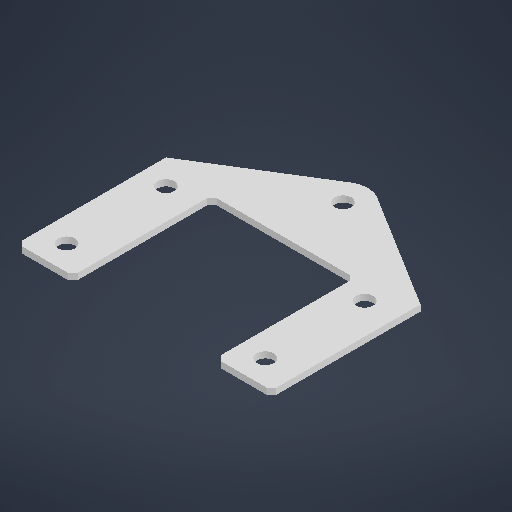
# Autodesk Inventor part: frontFunnel
Saved by Autodesk Inventor 2025.2 (Build 292293000, 293)
## iProperties
Created: 2025-03-23
Part Number: frontFunnel
Material: Generic
Document SubType Name: Modeling
Designer: Jahan
Density: 1 g/cm^3
Appearance: Default
Author: Jahan
Autodesk Inventor part; units mm, degrees
ref_plane "YZ Plane" through (0, 0, 0) normal (1, 0, 0) x (0, 1, 0)
ref_plane "XZ Plane" through (0, 0, 0) normal (0, 1, 0) x (-1, 0, 0)
ref_plane "XY Plane" through (0, 0, 0) normal (0, 0, 1) x (1, 0, 0)
sketch "Sketch1" plane through (0, 0, 0) normal (0, 1, 0) x (-1, 0, 0)
  circle A0 centre (21.6608, 3.3771) radius 2.1844
  circle A1 centre (21.6608, 28.7771) radius 2.1844
  circle A2 centre (-29.1392, 28.7771) radius 2.1844
  circle A3 centre (-29.1392, 3.3771) radius 2.1844
  line L0 (28.0108, 8.7873) -> (28.0108, -1.9569)
  line L1 (21.6608, 35.1271) -> (26.7408, 35.1271)
  line L2 (28.0108, 33.8571) -> (28.0108, -1.9569)
  line L3 (21.6608, 35.1271) -> (14.9933, 35.1271)
  line L4 (26.7408, 35.1271) -> (28.0108, 33.8571)
  line L5 (13.7233, 33.8571) -> (13.7233, 0.8371)
  line L6 (12.4533, -0.4329) -> (-21.5192, -0.4329)
  line L7 (14.9933, 35.1271) -> (13.7233, 33.8571)
  line L8 (13.7233, 0.8371) -> (12.4533, -0.4329)
  line L9 (-22.7892, 0.8371) -> (-22.7892, 33.8571)
  line L10 (-24.0592, 35.1271) -> (-35.8067, 35.1271)
  line L11 (-37.0767, 33.8571) -> (-37.0767, -2.9729)
  line L12 (-22.7892, 33.8571) -> (-24.0592, 35.1271)
  line L13 (-35.8067, 35.1271) -> (-37.0767, 33.8571)
  line L14 (-21.5192, -0.4329) -> (-22.7892, 0.8371)
  line L15 (28.0108, -1.9569) -> (28.0108, 3.3771)
  line L16 (21.6608, 3.3771) -> (47.0608, 3.3771) construction
  line L17 (-37.0767, -2.9729) -> (-7.8315, -21.1135)
  line L18 (28.0108, -1.9569) -> (28.0108, -2.9729)
  line L19 (28.0108, -2.9729) -> (-1.2009, -21.0641)
  arc A4 (-7.8315, -21.1135) -> (-1.2009, -21.0641) centre (-4.5565, -15.6732) ccw
  line L20 (28.0108, -2.9729) -> (-37.0767, -2.9729)
  line L21 (-4.5093, -22.023) -> (-4.5329, -2.9729)
  circle A5 centre (-4.5565, -15.6732) radius 2.1844
  point P0 (0, 0)
  point P1 (28.0108, 35.1271)
  point P2 (13.7233, 35.1271)
  point P3 (13.7233, -0.4329)
  point P4 (-22.7892, -0.4329)
  point P5 (-22.7892, 35.1271)
  point P6 (-37.0767, 35.1271)
  dimension "d0" = 6.35
  dimension "d1" = 1.27
  dimension "d2" = 1.27
  dimension "d3" = 35.56
  dimension "d4" = 1.27
  dimension "d5" = 1.27
  dimension "d6" = 1.27
  dimension "d7" = 1.27
  dimension "d8" = 35.56
  dimension "d9" = 1.27
  dimension "d10" = 1.27
  dimension "d11" = 1.27
  dimension "d12" = 1.27
  dimension "d13" = 1.27
  dimension "d14" = 1.27
  dimension "d18" = 6.35
  dimension "d19" = 1.016
  dimension "d20" = 36.83
  dimension "d21" = 4.3688
  constraints: 44 end point, 13 point on line, 6 centre point, 3 point on circle, 3 vertical, 2 horizontal, 2 perpendicular, 1 coincident, 1 collinear, 1 midpoint, 1 other
  measures "d0" distance of A1.centre L1.start
  measures "d1" distance of L1.end point (28.011, 35.127)
  measures "d2" distance of L2.start point (28.011, 35.127)
  measures "d3" distance of point (13.723, 35.127) point (13.723, -0.433)
  measures "d4" distance of L7.start point (13.723, 35.127)
  measures "d5" distance of L5.start point (13.723, 35.127)
  measures "d6" distance of L5.end point (13.723, -0.433)
  measures "d7" distance of L6.start point (13.723, -0.433)
  measures "d8" distance of point (-22.789, -0.433) point (-22.789, 35.127)
  measures "d9" distance of L9.end point (-22.789, 35.127)
  measures "d10" distance of L12.end point (-22.789, 35.127)
  measures "d11" distance of L13.start point (-37.077, 35.127)
  measures "d12" distance of L11.start point (-37.077, 35.127)
  measures "d13" distance of L14.start point (-22.789, -0.433)
  measures "d14" distance of L9.start point (-22.789, -0.433)
  measures "d18" radius of A4
  measures "d19" distance of L0.end L18.end
  measures "d20" distance of L11.start L11.end
  measures "d21" diameter of A5
extrude "Extrusion1" add sketch "Sketch1" along normal blind 1.5875 contours L0 L18 L20 L11 L13 L10 L12 L9 L14 L6 L8 L5 L7 L3 L1 L4 L2 | L19 A4 L21 A5 L20 | L21 A5 A4 L17 L20
equation "\"d5\" = d4"
equation "\"d6\" = d4"
equation "\"d7\" = d6"
equation "\"d10\" = d9"
equation "\"d11\" = d9"
equation "\"d12\" = d11"
equation "\"d13\" = d9"
equation "\"d14\" = d13"
body "Solid1"
